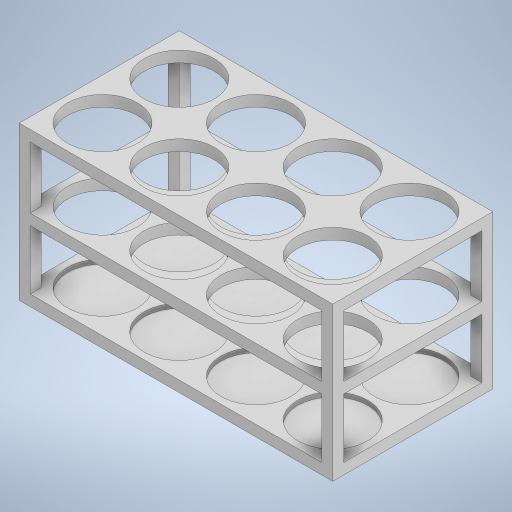
# Autodesk Inventor part: falcon tube mount v01
Saved by Autodesk Inventor 2023.5 (Build 275446000, 446)
## iProperties
Created: 2024-09-06
Part Number: falcon tube mount v01
Material: Generic
Document SubType Name: Modeling
Designer: Akramilab
Density: 1 g/cm^3
Appearance: Default
Author: Akramilab
Autodesk Inventor part; units mm, degrees
ref_plane "YZ Plane" through (0, 0, 0) normal (1, 0, 0) x (0, 1, 0)
ref_plane "XZ Plane" through (0, 0, 0) normal (0, 1, 0) x (-1, 0, 0)
ref_plane "XY Plane" through (0, 0, 0) normal (0, 0, 1) x (1, 0, 0)
sketch "Sketch1" plane through (0, 0, 0) normal (0, 1, 0) x (-1, 0, 0)
  line L0 (0, 0) -> (-143, 0)
  line L1 (-143, 0) -> (-143, 73)
  line L2 (-143, 73) -> (0, 73)
  line L3 (0, 73) -> (0, 0)
  line L4 (-38.5547, 3.9462) -> (-41.5547, 3.9462)
  circle A0 centre (-19, 19) radius 16
  circle A1 centre (-54, 19) radius 16
  circle A2 centre (-89, 19) radius 16
  circle A3 centre (-124, 19) radius 16
  circle A4 centre (-124, 54) radius 16
  circle A5 centre (-89, 54) radius 16
  circle A6 centre (-54, 54) radius 16
  circle A7 centre (-19, 54) radius 16
  dimension "d10" = 3
  dimension "d12" = 32
  dimension "d13" = 32
  dimension "d14" = 32
  dimension "d15" = 32
  dimension "d16" = 32
  dimension "d17" = 32
  dimension "d18" = 32
  dimension "d19" = 32
  dimension "d20" = 35
  dimension "d21" = 19
  dimension "d22" = 35
  dimension "d23" = 35
  dimension "d24" = 19
  dimension "d25" = 19
  dimension "d26" = 19
  dimension "d27" = 19
  dimension "d28" = 19
  dimension "d29" = 19
  dimension "d30" = 35
  dimension "d31" = 35
  dimension "d32" = 35
  dimension "d33" = 35
  dimension "d34" = 19
  constraints: 10 end point, 8 centre point, 8 coincident, 2 horizontal, 2 parallel, 1 perpendicular
  measures "d10" distance of L4.start L4.end
  measures "d12" diameter of A0
  measures "d13" diameter of A1
  measures "d14" diameter of A2
  measures "d15" diameter of A3
  measures "d16" diameter of A7
  measures "d17" diameter of A6
  measures "d18" diameter of A5
  measures "d19" diameter of A4
  measures "d20" distance of A1.centre A0.centre
  measures "d21" distance from line of L3 A0.centre
  measures "d22" distance of A2.centre A1.centre
  measures "d23" distance of A3.centre point (-89, 19)
  measures "d24" distance from line of L1 A3.centre
  measures "d25" distance from line of L0 A0.centre
  measures "d26" distance from line of L3 A7.centre
  measures "d27" distance from line of L2 A7.centre
  measures "d28" distance from line of L2 A6.centre
  measures "d29" distance from line of L2 point (-89, 54)
  measures "d30" distance of A6.centre A7.centre
  measures "d31" distance of point (-89, 54) A6.centre
  measures "d32" distance of A4.centre A5.centre
  measures "d33" distance of point (-19, 54) A0.centre
  measures "d34" distance from line of L2 A4.centre
extrude "Extrusion1" add sketch "Sketch1" against normal blind 70
sketch "Sketch3" plane through (143, 0, 0) normal (0, 0, -1) x (-1, 0, 0)
  line L0 (138, -65) -> (5, -65)
  line L1 (5, -65) -> (5, -38)
  line L2 (5, -38) -> (138, -38)
  line L3 (138, -38) -> (138, -65)
  line L4 (143, 0) -> (143, -70) projected
  line L5 (0, 0) -> (0, -70) projected
  line L6 (143, -70) -> (0, -70) projected
  line L7 (0, 0) -> (143, 0) projected
  line L8 (5, -5) -> (138, -5)
  line L9 (138, -5) -> (138, -33)
  line L10 (138, -33) -> (5, -33)
  line L11 (5, -33) -> (5, -5)
  line L12 (5, -5) -> (138, -33) construction
  line L13 (138, -5) -> (5, -33) construction
  point P0 (71.5, -19)
  dimension "d37" = 5
  dimension "d38" = 5
  dimension "d39" = 5
  dimension "d57" = 5
  dimension "d58" = 5
  dimension "d59" = 5
  dimension "d63" = 5
  constraints: 20 end point, 4 parallel, 2 horizontal, 2 midpoint, 2 perpendicular
  measures "d37" distance between parallel lines of L4 L3
  measures "d38" distance between parallel lines of L5 L1
  measures "d39" distance between parallel lines of L0 L6
  measures "d57" distance between parallel lines of L7 L8
  measures "d58" distance between parallel lines of L5 L11
  measures "d59" distance between parallel lines of L4 L9
  measures "d63" distance between parallel lines of L2 L10
extrude "Extrusion2" cut sketch "Sketch3" against normal through all contours L0 L1 L2 L3 | L8 L9 L10 L11
sketch "Sketch4" plane through (0, 0, 0) normal (-1, 0, 0) x (0, 0, 1)
  line L0 (5, -5) -> (68, -5)
  line L1 (68, -5) -> (68, -33)
  line L2 (68, -33) -> (5, -33)
  line L3 (5, -33) -> (5, -5)
  line L4 (0, 0) -> (73, 0) projected
  line L5 (0, 0) -> (0, -70) projected
  line L6 (73, 0) -> (73, -70) projected
  line L7 (5, -38) -> (68, -38)
  line L8 (68, -38) -> (68, -65)
  line L9 (68, -65) -> (5, -65)
  line L10 (5, -65) -> (5, -38)
  line L11 (73, -70) -> (0, -70) projected
  dimension "d45" = 5
  dimension "d46" = 5
  dimension "d47" = 5
  dimension "d49" = 5
  dimension "d50" = 5
  dimension "d51" = 5
  dimension "d62" = 5
  constraints: 16 end point, 4 parallel, 2 horizontal, 2 perpendicular
  measures "d45" distance between parallel lines of L0 L4
  measures "d46" distance between parallel lines of L5 L3
  measures "d47" distance between parallel lines of L6 L1
  measures "d49" distance between parallel lines of L9 L11
  measures "d50" distance between parallel lines of L6 L8
  measures "d51" distance between parallel lines of L5 L10
  measures "d62" distance between parallel lines of L7 L2
extrude "Extrusion3" cut sketch "Sketch4" against normal through all contours L0 L1 L2 L3 | L7 L8 L9 L10
sketch "Sketch5" plane through (0, -70, 0) normal (0, -1, 0) x (1, 0, 0)
  line L0 (143, 0) -> (0, 0) projected
  line L1 (143, 0) -> (0, 0)
  line L2 (0, 0) -> (0, 73)
  line L3 (0, 73) -> (143, 73)
  line L4 (143, 73) -> (143, 0)
  constraints: 8 end point, 2 parallel, 1 horizontal, 1 perpendicular
extrude "Extrusion4" add sketch "Sketch5" against normal blind 3
equation "\"d13\" = d12"
equation "\"d14\" = d12"
equation "\"d15\" = d12"
equation "\"d16\" = d12"
equation "\"d17\" = d12"
equation "\"d18\" = d12"
equation "\"d19\" = d12"
equation "\"d20\" = d12 + d10"
equation "\"d21\" = 0.5 * d12 + d10"
equation "\"d22\" = d20"
equation "\"d23\" = d22"
equation "\"d24\" = d21"
equation "\"d25\" = d21"
equation "\"d26\" = d21"
equation "\"d27\" = d25"
equation "\"d28\" = d27"
equation "\"d29\" = d27"
equation "\"d30\" = d20"
equation "\"d31\" = d30"
equation "\"d32\" = d31"
equation "\"d33\" = d20"
equation "\"d34\" = d29"
equation "\"d38\" = d37"
equation "\"d39\" = d37"
equation "\"d57\" = d37"
equation "\"d58\" = d38"
equation "\"d59\" = d37"
equation "\"d63\" = d37"
equation "\"d46\" = d45"
equation "\"d47\" = d45"
equation "\"d49\" = d45"
equation "\"d50\" = d45"
equation "\"d51\" = d45"
equation "\"d62\" = d45"
body "Solid1"
